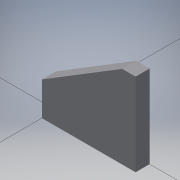
# Autodesk Inventor part: Лепесток
Saved by Autodesk Inventor 2019 (Build 230136000, 136)
## iProperties
Created: 2022-06-28
Part Number: Лепесток
Material: Типовые
Document SubType Name: Modeling
Designer: korsh
Density: 1 g/cm^3
Appearance: По умолчанию
Author: korsh
Autodesk Inventor part; units mm, degrees
ref_plane "YZ Plane" through (0, 0, 0) normal (1, 0, 0) x (0, 1, 0)
ref_plane "XZ Plane" through (0, 0, 0) normal (0, 1, 0) x (-1, 0, 0)
ref_plane "XY Plane" through (0, 0, 0) normal (0, 0, 1) x (1, 0, 0)
sketch "Эскиз1" plane through (0, 0, 0) normal (0, 0, 1) x (1, 0, 0)
  line L0 (40, 0) -> (0, 0) projected
  line L1 (40, 0) -> (40, -6) projected
  line L2 (0, -6) -> (40, -6) projected
  line L3 (0, 0) -> (0, -6) projected
  line L4 (0, 0) -> (0, 20)
  line L5 (0, 20) -> (18.33, 29.326)
  line L6 (40, 0) -> (40, 29.326)
  line L7 (40, 29.326) -> (18.33, 29.326)
  dimension "d0" = 20
  constraints: 8 end point, 2 vertical, 1 perpendicular
  measures "d0" distance of L0.end L4.end
extrude "Выдавливание1" add sketch "Эскиз1" along normal blind 6
sketch "Эскиз2" plane through (0, 0, 6) normal (0, 0, 1) x (1, 0, 0)
  line L0 (0, 20) -> (0, -6) projected
  line L1 (40, 29.326) -> (18.33, 29.326) projected
  line L2 (18.33, 29.326) -> (0, 20)
  line L3 (18.33, 29.326) -> (0, 20) projected
  line L4 (0, 8.2778) -> (18.33, 29.326)
  point P0 (0, 0)
  constraints: 4 end point, 1 point on line
extrude "Выдавливание2" cut sketch "Эскиз2" against normal blind 6
sketch "Эскиз3" plane through (0, 0, 6) normal (0, 0, 1) x (1, 0, 0)
  line L0 (0, 8.2778) -> (0, -6) projected
  line L1 (0, 8.2778) -> (34.2751, 29.326)
  line L2 (40, 29.326) -> (18.33, 29.326) projected
  line L3 (0, 8.2778) -> (18.33, 29.326)
  line L4 (18.33, 29.326) -> (34.2751, 29.326)
  point P0 (0, 0)
  constraints: 6 end point, 1 collinear, 1 point on line
extrude "Выдавливание3" cut sketch "Эскиз3" against normal blind 6
sketch "Эскиз4" plane through (0, 0, 0) normal (0, 0, -1) x (-1, 0, 0)
  point P0 (0, 0)
sketch "Эскиз5" plane through (0, 0, 0) normal (0, 0, -1) x (-1, 0, 0)
  line L0 (4.9019, -6) -> (-15.0981, -6) projected
  line L1 (0, -6) -> (-40, -6) projected
  point P0 (0, 0)
